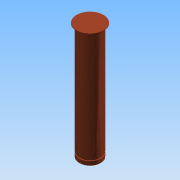
# Autodesk Inventor part: 皮带轮轴
Saved by Autodesk Inventor 2015 (Build 190159000, 159)
## iProperties
Created: 2017-05-28
Part Number: 皮带轮轴
Material: 常规
Document SubType Name: Modeling
Designer: Administrator
Density: 1 g/cm^3
Appearance: 铜 - 缎光
Author: Administrator
Autodesk Inventor part; units mm, degrees
ref_plane "YZ Plane" through (0, 0, 0) normal (1, 0, 0) x (0, 1, 0)
ref_plane "XZ Plane" through (0, 0, 0) normal (0, 1, 0) x (-1, 0, 0)
ref_plane "XY Plane" through (0, 0, 0) normal (0, 0, 1) x (1, 0, 0)
sketch "草图1" plane through (0, 0, 0) normal (0, 0, 1) x (1, 0, 0)
  circle A0 centre (0, 0) radius 10
  dimension "d0" = 20
  constraints: 1 centre point, 1 coincident
  measures "d0" diameter of A0
extrude "拉伸1" add sketch "草图1" along normal blind 108.34
sketch "草图2" plane through (0, 0, 108.34) normal (0, 0, 1) x (1, 0, 0)
  circle A0 centre (0, 0) radius 12.5
  dimension "d3" = 25
  constraints: 1 centre point, 1 coincident
  measures "d3" diameter of A0
extrude "拉伸2" add sketch "草图2" against normal blind 0.6
sketch "草图3" plane through (0, 0, 0) normal (0, 1, 0) x (-1, 0, 0)
  line L0 (15.328, 4) -> (9.175, 4)
  line L1 (9.175, 4) -> (9.175, 5.2)
  line L2 (9.175, 5.2) -> (15.328, 5.2)
  line L3 (15.328, 5.2) -> (15.328, 4)
  line L4 (0, 0) -> (0, -10.7224)
  line L5 (-10, 0) -> (10, 0) projected
  dimension "d6" = 10.7224
  dimension "d7" = 1.2
  dimension "d8" = 4
  dimension "d9" = 9.175
  dimension "d10" = 6.153
  constraints: 10 end point, 2 parallel, 1 horizontal, 1 perpendicular, 1 vertical
  measures "d6" distance of L4.start L4.end
  measures "d7" distance of L2.end L0.start
  measures "d8" distance between parallel lines of L5 L0
  measures "d9" distance between parallel lines of L4 L1
  measures "d10" distance of L1.end L2.end
revolve "旋转1" cut sketch "草图3" angle 360 about axis through (0, 0, 0) along (0, 0, -1)
chamfer "倒角1" distance 0.5 angle 45 1 edges at (-10, 0, 0)
